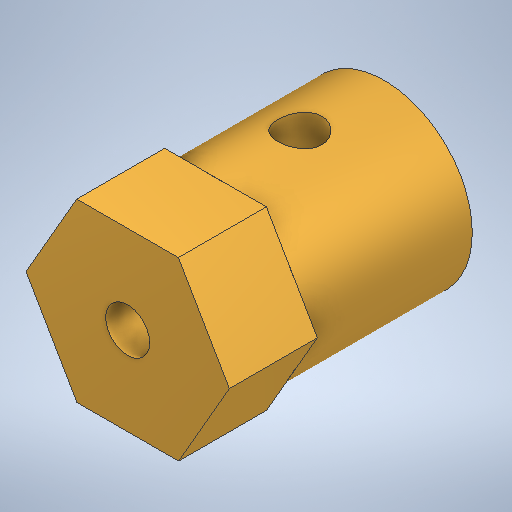
# Autodesk Inventor part: Wheel Test
Saved by Autodesk Inventor 2025.2 (Build 292293000, 293)
## iProperties
Created: 2025-01-16
Part Number: Wheel Test
Material: Generic
Document SubType Name: Modeling
Designer: Matt Tidd
Density: 1 g/cm^3
Appearance: Default
Author: Matt Tidd
Autodesk Inventor part; units mm, degrees
ref_plane "YZ Plane" through (0, 0, 0) normal (1, 0, 0) x (0, 1, 0)
ref_plane "XZ Plane" through (0, 0, 0) normal (0, 1, 0) x (-1, 0, 0)
ref_plane "XY Plane" through (0, 0, 0) normal (0, 0, 1) x (1, 0, 0)
sketch "Sketch2" plane through (0, 0, 0) normal (0, 0, 1) x (1, 0, 0)
  circle A0 centre (0, 0) radius 6
  dimension "d3" = 12
  constraints: 1 centre point, 1 coincident
  measures "d3" diameter of A0
extrude "Extrusion2" add sketch "Sketch2" along normal blind 11.5
sketch "Sketch3" plane through (0, 0, 11.5) normal (0, 0, 1) x (1, 0, 0)
  line L0 (-3.476, 6) -> (3.4581, 6.0103)
  line L1 (3.4581, 6.0103) -> (6.9342, 0.0103)
  line L2 (6.9342, 0.0103) -> (3.476, -6)
  line L3 (3.476, -6) -> (-3.4581, -6.0103)
  line L4 (-3.4581, -6.0103) -> (-6.9342, -0.0103)
  line L5 (-6.9342, -0.0103) -> (-3.476, 6)
  point P0 (0, 0)
  point P1 (0, 0)
  constraints: 12 end point, 1 coincident, 13 other
sketch "Sketch4" plane through (0, 0, 0) normal (0, 0, -1) x (-1, 0, 0)
  circle A0 centre (0, 0) radius 3
  dimension "d6" = 6
  constraints: 1 centre point, 1 coincident
  measures "d6" diameter of A0
extrude "Extrusion3" add sketch "Sketch3" along normal blind 6
extrude "Extrusion4" cut sketch "Sketch4" against normal up to surface (11.5 mm away)
sketch "Sketch5" plane through (-3.476, 6, 17.5) normal (-0.0014906, 0.9999989, 0) x (0.9999989, 0.0014906, 0)
  line L0 (0, 0) -> (-3.4671, 0) projected
  line L1 (6.9342, 6) -> (6.9342, 0) projected
  line L2 (0, 0) -> (6.9342, 0)
  line L3 (6.9342, 0) -> (6.9342, 6)
  line L4 (6.9342, 6) -> (0, 6)
  line L5 (0, 6) -> (0, 0)
  line L6 (3.4671, 0) -> (3.4671, 17.5) construction
  line L7 (6.9342, 6) -> (0, 6) construction
  line L8 (6.9342, 6) -> (0, 6) construction
  circle A0 centre (3.4671, 11.75) radius 1.5
  dimension "d11" = 3
  constraints: 12 end point, 3 equal length, 1 centre point, 1 coincident, 1 horizontal, 1 midpoint, 1 perpendicular, 1 point on line, 1 vertical
  measures "d11" diameter of A0
extrude "Extrusion5" cut sketch "Sketch5" against normal through all contours A0
sketch "Sketch6" plane through (0, 0, 17.5) normal (0, 0, 1) x (1, 0, 0)
  circle A0 centre (0, 0) radius 1.5
  dimension "d14" = 3
  constraints: 1 centre point, 1 coincident
  measures "d14" diameter of A0
extrude "Extrusion6" cut sketch "Sketch6" against normal blind 10
body "Solid2"
